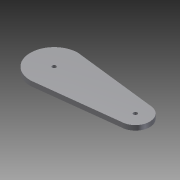
# Autodesk Inventor part: short arm
Saved by Autodesk Inventor 2011 (Build 150239000, 239)
## iProperties
Created: 2010-04-19
Part Number: short arm
Document SubType Name: Modeling
Designer: lucio
Density: 1 g/cm^3
Mass: 166.806 g
Surface Area: 416.956 cm^2
Volume: 166.806 cm^3
Author: lucio
Autodesk Inventor part; units mm, degrees
ref_plane "YZ Plane" through (0, 0, 0) normal (1, 0, 0) x (0, 1, 0)
ref_plane "XZ Plane" through (0, 0, 0) normal (0, 1, 0) x (-1, 0, 0)
ref_plane "XY Plane" through (0, 0, 0) normal (0, 0, 1) x (1, 0, 0)
sketch "Sketch1" plane through (0, 0, 0) normal (0, 0, 1) x (1, 0, 0)
  circle A0 centre (78.9796, 4.5334) radius 50
  circle A1 centre (248.9796, 4.5334) radius 30
  line L0 (78.9796, 54.5334) -> (248.9796, 34.5334)
  line L1 (248.9796, -25.4666) -> (78.9796, -45.4666)
  dimension "d25" = 170
  dimension "d26" = 100
  dimension "d27" = 60
  dimension "d28" = 0
  constraints: 4 end point, 4 point on circle, 2 centre point
  measures "d25" distance of A1.centre A0.centre
  measures "d26" diameter of A0
  measures "d27" diameter of A1
  measures "d28" vertical distance of A1.centre A0.centre
extrude "Extrusion1" add sketch "Sketch1" along normal blind 10 contours L0 A0 L1 | L0 A1 L1 A0 | A1
sketch "Sketch2" plane through (0, 0, 10) normal (0, 0, 1) x (1, 0, 0)
  arc A0 (248.9796, -25.4666) -> (248.9796, 34.5334) centre (248.9796, 4.5334) ccw projected
  arc A1 (78.9796, 54.5334) -> (78.9796, -45.4666) centre (78.9796, 4.5334) ccw projected
  constraints: 2 coincident
hole "Hole1" at (78.9796, 4.5334, 10) at (248.9796, 4.5334, 10) direction (0, 0, -1) diameter 8 end through all
body "Solid1"
